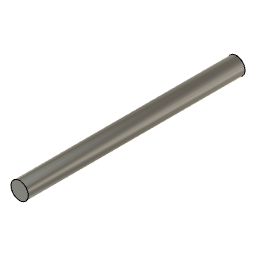
assembly v8 (Autodesk Fusion 360 archive; units mm, degrees)
design "rod"
Autodesk Fusion 360 part; units mm, degrees
sketch "Sketch1" plane through (0, 0, 0) normal (0, 1, 0) x (1, 0, 0)
  circle A0 centre (0, 0) radius 2
  dimension "d1" = 4
  constraint coincident A0.centre origin
  measures "d1" diameter of A0
extrude "Extrude1" add sketch "Sketch1" along normal blind 50

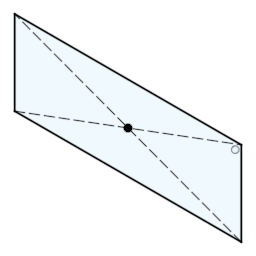
design "door"
Autodesk Fusion 360 part; units mm, degrees
sketch "Sketch1" plane through (0, 0, 0) normal (0, 1, 0) x (1, 0, 0)
  line L0 (87.5, 32.5) -> (-87.5, 32.5)
  line L1 (-87.5, 32.5) -> (-87.5, -32.5)
  line L2 (-87.5, -32.5) -> (87.5, -32.5)
  line L3 (87.5, -32.5) -> (87.5, 32.5)
  line L4 (87.5, 32.5) -> (-87.5, -32.5) construction
  line L5 (-87.5, 32.5) -> (87.5, -32.5) construction
  circle A0 centre (82.7907, -26.8724) radius 1.5
  dimension "d1" = 175
  dimension "d2" = 65
  dimension "d5" = 3
  constraint horizontal L0
  constraint perpendicular L0 L1
  constraint parallel L0 L2
  constraint parallel L1 L3
  constraint coincident L4 origin
  constraint coincident L5 origin
  measures "d1" distance of L1.end L2.end
  measures "d2" distance of L0.end L1.end
  measures "d5" diameter of A0
extrude "Extrude1" add sketch "Sketch1" along normal blind 5 contours L0 L1 L2 L3 | A0

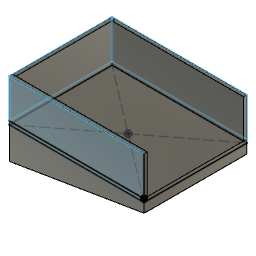
design "trolley"
Autodesk Fusion 360 part; units mm, degrees
sketch "Sketch1" plane through (0, 0, 0) normal (0, 0, 1) x (1, 0, 0)
  line L0 (105, -80) -> (-105, -80)
  line L1 (-105, -80) -> (-105, 80)
  line L2 (-105, 80) -> (105, 80)
  line L3 (105, 80) -> (105, -80)
  line L4 (105, -80) -> (-105, 80) construction
  line L5 (-105, -80) -> (105, 80) construction
  dimension "d1" = 210
  dimension "d2" = 160
  constraint horizontal L0
  constraint perpendicular L0 L1
  constraint parallel L0 L2
  constraint parallel L1 L3
  constraint coincident L4 origin
  constraint coincident L5 origin
  measures "d1" distance of L1.end L2.end
  measures "d2" distance of L0.end L1.end
extrude "Extrude1" add sketch "Sketch1" along normal blind 5
ref_plane "WorkPlane1" through (0, 80, 0) normal (0, 1, 0) x (0, 0, 1)
ref_plane "WorkPlane2" through (0, -80, 0) normal (0, 1, 0) x (0, 0, 1)
sketch "Sketch2" plane through (0, -80, 0) normal (0, 1, 0) x (1, 0, 0)
sketch "Sketch3" plane through (0, 80, 0) normal (0, 1, 0) x (1, 0, 0)
  line L0 (104.9931, -4.7484) -> (-105.257, -4.7484)
  line L1 (-105.257, -4.7484) -> (-105.257, -64.8953)
  line L2 (-105.257, -64.8953) -> (104.9931, -64.8953)
  line L3 (104.9931, -64.8953) -> (104.9931, -4.7484)
  constraint horizontal L0
  constraint vertical L1
  constraint horizontal L2
  constraint vertical L3
ref_plane "WorkPlane3" through (-105, 0, 0) normal (1, 0, 0) x (0, 1, 0)
sketch "Sketch4" plane through (-105, 0, 0) normal (1, 0, 0) x (0, 1, 0)
  line L0 (80, 65) -> (-80, 65)
  line L1 (-80, 65) -> (-80, 5)
  line L2 (-80, 5) -> (80, 5)
  line L3 (80, 5) -> (80, 65)
  constraint horizontal L0
  constraint vertical L1
  constraint horizontal L2
  constraint vertical L3
sketch "Sketch5" plane through (0, -80, 0) normal (0, -1, 0) x (1, 0, 0)
  line L0 (-105, 0) -> (105, 0)
  line L1 (105, 0) -> (105, 5)
  line L2 (105, 5) -> (-105, 5)
  line L3 (-105, 5) -> (-105, 0)
  line L4 (-105, 65.4104) -> (105, 65.4104)
  line L5 (105, 65.4104) -> (105, 5)
  line L6 (105, 5) -> (-105, 5)
  line L7 (-105, 5) -> (-105, 65.4104)
  constraint horizontal L4
  constraint vertical L5
  constraint horizontal L6
  constraint vertical L7
  constraint coincident L1.end L2.start
sketch "Sketch6" plane through (-0.1319, 80, 34.8218) normal (0, 1, 0) x (1, 0, 0)
extrude "Extrude2" add sketch "Sketch3" against normal blind 5
extrude "Extrude3" add sketch "Sketch4" along normal blind 5
extrude "Extrude4" add sketch "Sketch5" against normal blind 5 contours L2 L4 L5 L6 L7
sketch "Sketch7" plane through (0, -80, 0) normal (0, -1, 0) x (1, 0, 0)
  line L0 (-105, 65.4104) -> (-105, 0)
  line L1 (-105, 0) -> (105, 0)
  line L2 (105, 0) -> (105, 65.4104)
  line L3 (105, 65.4104) -> (-105, 65.4104)
sketch "Sketch8" plane through (0, -80, 0) normal (0, -1, 0) x (1, 0, 0)
  line L0 (-105, -50) -> (105, -15)
  line L1 (105, 0) -> (105, -15)
  constraint vertical L1
sketch "Sketch9" plane through (0, -80, 0) normal (0, -1, 0) x (1, 0, 0)
  line L0 (-105, 0) -> (105, 0)
  constraint horizontal L0
sketch "Sketch10" plane through (0, -80, 0) normal (0, -1, 0) x (1, 0, 0)
  line L0 (-105, 0) -> (-105, -50)
  constraint vertical L0
sketch "Sketch11" plane through (0, 80, 0) normal (0, 1, 0) x (1, 0, 0)
  line L0 (-105, 0) -> (-105, 50)
  line L1 (-105, 50) -> (105, 15)
  line L2 (105, 15) -> (105, 0)
  line L3 (105, 0) -> (-105, 0)
  constraint vertical L0
  constraint parallel L0 L2
  constraint perpendicular L0 L3
sketch "Sketch12" plane through (0, -80, 35.2052) normal (0, -1, 0) x (1, 0, 0)
  line L0 (-105, -35) -> (-105, -85)
  line L1 (-105, -85) -> (105, -50)
  line L2 (105, -50) -> (105, -35)
  line L3 (105, -35) -> (-105, -35)
  constraint vertical L0
  constraint parallel L0 L2
  constraint perpendicular L0 L3
extrude "Extrude5" add sketch "Sketch11" against normal blind 5
extrude "Extrude6" add sketch "Sketch12" against normal blind 5
sketch "Sketch13" plane through (-105, 0, 0) normal (1, 0, 0) x (0, 1, 0)
  line L0 (75, -50) -> (-75, -50)
  line L1 (-75, -50) -> (-75, 0)
  line L2 (-75, 0) -> (75, 0)
  line L3 (75, 0) -> (75, -50)
  constraint horizontal L0
  constraint perpendicular L0 L1
  constraint perpendicular L1 L2
  constraint perpendicular L0 L3
extrude "Extrude7" add sketch "Sketch13" along normal blind 5
sketch "Sketch14" plane through (105, 0, 0) normal (1, 0, 0) x (0, 1, 0)
  line L0 (-80, 65.4104) -> (-80, -14.7948)
  line L1 (-80, -14.7948) -> (-75, -14.7948)
  line L2 (-75, -14.7948) -> (-75, 0)
  line L3 (-75, 0) -> (75, 0)
  line L4 (75, 0) -> (75, -15)
  line L5 (75, -15) -> (80, -15)
  line L6 (80, -15) -> (80, 5)
  line L7 (80, 5) -> (-75, 5)
  line L8 (-75, 5) -> (-75, 65.4104)
  line L9 (-75, 65.4104) -> (-80, 65.4104)
  line L10 (-75, 0) -> (75, 0)
  line L11 (75, 0) -> (75, -15)
  line L12 (75, -15) -> (-75, -15)
  line L13 (-75, -15) -> (-75, 0)
  constraint horizontal L10
  constraint vertical L11
  constraint horizontal L12
  constraint vertical L13
  constraint coincident L4.end L5.start
  constraint coincident L2.end L3.start
extrude "Extrude8" add sketch "Sketch14" against normal blind 5 contours L2 L3 L4 L10 L11 L12 L13
